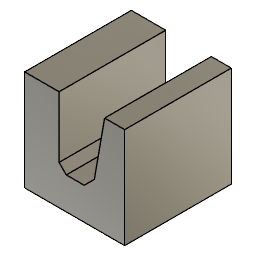
Cutting Block Femoral Shell (L&R) (Autodesk Fusion 360 design; units mm, degrees)
Autodesk Fusion 360 part; units mm, degrees
sketch "Sketch1" plane through (0, 0, 0) normal (0, 1, 0) x (1, 0, 0)
  line L0 (13.25, 0) -> (-13.25, 0)
  line L1 (13.25, 0) -> (28.25, -15)
  line L2 (-13.25, 0) -> (-23.85, -10.6)
  line L3 (28.25, -15) -> (36.0642, -59.3163)
  line L4 (-23.85, -10.6) -> (-23.85, -26.6)
  line L5 (0, 0) -> (0, -16) construction
  circle A0 centre (-13.85, -13) radius 16.8808
  line L6 (0, -16) -> (2.9008, -16)
  line L7 (2.9008, -16) -> (3.9843, 0) construction
  line L8 (0, 23.4514) -> (0, -71.5486) construction
  line L9 (-55, 9) -> (76.6583, 9) construction
  line L10 (40.3824, -55.0125) -> (29.0953, 9) construction
  line L11 (-32.85, -64.9999) -> (-32.85, 12.841) construction
  circle A1 centre (-0.9196, -26.7704) radius 35.7704
  circle A2 centre (-68.0139, -44.3984) radius 105.1418
  line L12 (74.0804, 48.6) -> (-75.9196, 48.6)
  line L13 (-75.9196, 48.6) -> (-75.9196, -102.1408)
  line L14 (-75.9196, -102.1408) -> (74.0804, -102.1408)
  line L15 (74.0804, -102.1408) -> (74.0804, 48.6)
  line L16 (74.0804, 48.6) -> (-75.9196, -102.1408) construction
  line L17 (-75.9196, 48.6) -> (74.0804, -102.1408) construction
  line L18 (-23.85, -26.6) -> (-75.9196, -26.7704)
  line L19 (34.8508, -26.7704) -> (74.0804, -26.7704)
  line L20 (36.0642, -59.3163) -> (43.6153, -102.1408)
  line L21 (-23.85, -26.6) -> (-23.85, -102.1408)
  point P0 (-0.9196, -26.7704)
  dimension "d1" = 26.5
  dimension "d2" = 135
  dimension "d3" = 135
  dimension "d5" = 15
  dimension "d7" = 16
  dimension "d8" = 16
  dimension "d10" = 9
  dimension "d11" = 5
  dimension "d12" = 9
  dimension "d13" = 10
  dimension "d14" = 13
  dimension "d15" = 65
  dimension "d59" = 45
  dimension "d60" = 145
  dimension "d62" = 10.6
  dimension "d121" = 150
  dimension "d131" = 39.6
  constraint horizontal L0
  constraint midpoint L5.start L0
  constraint vertical L4
  constraint coincident L5.start origin
  constraint perpendicular L0 L5
  constraint coincident L4.end A0
  constraint perpendicular L5 L6
  constraint coincident L0 L7.end
  constraint perpendicular L0 L8
  constraint parallel L0 L9
  constraint parallel L3 L10
  constraint perpendicular L9 L11
  constraint coincident L5.start L8
  constraint coincident L9 L10.end
  constraint tangent L10 A1
  constraint tangent L9 A1
  constraint tangent A0 A1
  constraint tangent A1 A2
  constraint coincident L3.end A2
  constraint horizontal L12
  constraint perpendicular L12 L13
  constraint parallel L12 L14
  constraint parallel L13 L15
  constraint coincident L16 P0
  constraint coincident L17 P0
  constraint coincident P0 A1.centre
  constraint midpoint L13 L18.end
  constraint coincident A1 L19.start
  constraint midpoint L15 L19.end
  constraint perpendicular L15 L19
  constraint coincident L14 L20.end
  constraint collinear L3 L20
  constraint coincident L14 L21.end
  constraint perpendicular L14 L21
  measures "d1" distance of L0.start L0.end
  measures "d2" angle of L0 L2
  measures "d3" angle of L0 L1
  measures "d5" horizontal distance of L0.start L1.end
  measures "d7" distance of L2.end L4.end
  measures "d8" distance of L5.start L5.end
  measures "d10" distance of L0 L9
  measures "d11" distance of L3 L10
  measures "d12" distance of L4 L11
  measures "d13" distance of L4 A0.centre
  measures "d14" distance of L0 A0.centre
  measures "d15" distance of L10.start L10.end
  measures "d59" distance of L1.end L3.end
  measures "d60" angle of L1 L3
  measures "d62" distance of L0.end L4
  measures "d121" distance of L12.start L12.end
  measures "d131" distance of L9 L12
extrude "Extrude1" add sketch "Sketch1" along normal mid plane 160 contours L0 L1 L3 A0 A1 | L0 L2 L4 A0 | A1 A2 L12 L13 L18 | A0 A1 L18 | L3 A1 A2 L19 | A1 L18 L21 | A1 A2 L19 | A2 L12 L15 L19 | A1 L13 L14 L18 L21 | A2 L14 L15 L19 L20 picked at (-20.2039, -3.2526)
move_face "OffsetFaces1" offset -0.4 5 faces at (-4.4167, 26.6667, 0) (-16.7833, -26.6667, 3.5333) (23.25, 26.6667, 10) (38.4935, 26.6667, 73.0938) (-23.85, -26.6667, 41.1136)
sketch "Sketch12" plane through (0, 0, -0.4) normal (0, 0, 1) x (-1, 0, 0)
  line L0 (13.4157, -80) -> (13.4157, 80)
  line L1 (13.4157, 80) -> (-13.4157, 80)
  line L2 (-13.4157, 80) -> (-13.4157, -80)
  line L3 (-13.4157, -80) -> (13.4157, -80)
  line L4 (0, -80) -> (0, 80) construction
  circle A0 centre (0, 25) radius 4.5
  line L5 (13.4157, 0) -> (-13.4157, 0)
  circle A1 centre (0, -25) radius 4.5
  dimension "d122" = 9
  dimension "d123" = 25
  constraint midpoint L3 L4.start
  constraint midpoint L1 L4.end
  constraint coincident L4 A0.centre
  constraint midpoint L0 L5.start
  constraint midpoint L2 L5.end
  constraint symmetric A0 L5 A1
  measures "d122" diameter of A0
  measures "d123" distance of origin A0.centre
ref_plane "WorkPlane3" through (0, -25, 15.6) normal (0, 0, 1) x (-1, 0, 0)
sketch "Sketch13" plane through (0, 0, 15.6) normal (0, 0, 1) x (1, 0, 0)
  circle A0 centre (0, -25) radius 3
  circle A1 centre (0, -25) radius 4.5
  line L0 (0, 0) -> (30, 0) construction
  circle A2 centre (0, 25) radius 3
  dimension "d125" = 6
  constraint concentric A0 A1
  constraint coincident L0.start origin
  constraint horizontal L0
  constraint symmetric A0 L0 A2
  measures "d125" diameter of A0
loft "Loft2" add profiles "Sketch12", "Sketch13" section 1 contours A0 section 2 contours A0
mirror "Mirror2" about plane through (0, 0, 0) normal (0, 1, 0) of "Loft2"
fillet "Fillet8" radius 2 2 edges at (-2.797, 23.9152, 15.6) (-2.797, -23.9152, 15.6)
